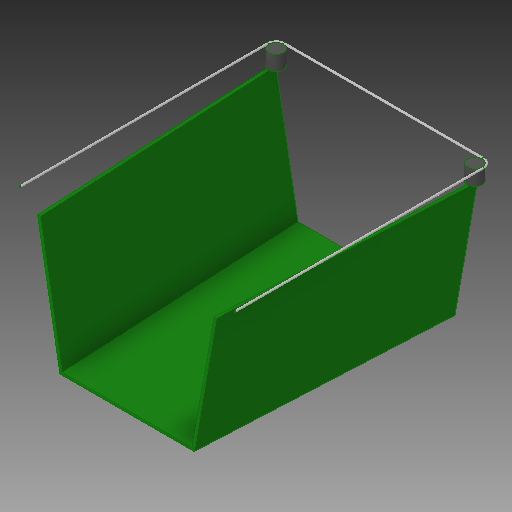
# Autodesk Inventor part: boat_segment
Saved by Autodesk Inventor 2019 (Build 230136000, 136)
## iProperties
Created: 2019-01-30
Part Number: boat_segment
Material: Generic
Document SubType Name: Modeling
Designer: suchanek
Density: 1 g/cm^3
Appearance: Default
boat_rim_angle: 80.00 deg
boat_width: 400.000 mm
boat_rim_thickness: 5.000 mm
boat_rim_plate_width: 0.000 mm
boat_part_length: 500.000 mm
boat_end_width: 350.000 mm
Author: suchanek
Autodesk Inventor part; units mm, degrees
ref_plane "YZ Plane" through (0, 0, 0) normal (1, 0, 0) x (0, 1, 0)
ref_plane "XZ Plane" through (0, 0, 0) normal (0, 1, 0) x (-1, 0, 0)
ref_plane "XY Plane" through (0, 0, 0) normal (0, 0, 1) x (1, 0, 0)
sketch "Sketch1" plane through (0, 0, 0) normal (0, 0, 1) x (1, 0, 0)
  line L0 (-160.1138, -255) -> (160.1138, -255)
  line L1 (200, 0) -> (155.9183, -250)
  line L2 (155.9183, -250) -> (-155.9183, -250)
  line L3 (-155.9183, -250) -> (-200, 0)
  line L4 (-160.1138, -255) -> (-204.1955, -5)
  line L5 (-204.1955, -5) -> (-204.1955, -5)
  line L6 (-204.1955, -5) -> (-205.0771, 0)
  line L7 (160.1138, -255) -> (204.1955, -5)
  line L8 (204.1955, -5) -> (204.1955, -5)
  line L9 (204.1955, -5) -> (205.0771, 0)
  line L10 (-205.0771, 0) -> (-200, 0)
  line L11 (200, 0) -> (205.0771, 0)
  line L12 (0, 0) -> (0, 16.0909)
  dimension "d0" = 5
  dimension "d1" = 5
  dimension "d2" = 5
  dimension "d3" = 0
  dimension "d4" = 0
  dimension "d5" = 400
  dimension "d6" = 250
  dimension "d7" = 80
  dimension "d8" = 80
  dimension "d9" = 5
  dimension "d10" = 5
  constraints: 26 end point, 4 horizontal, 3 collinear, 2 parallel, 1 horizontal alignment, 1 symmetric about line, 1 vertical
  measures "d0" distance between parallel lines of L2 L0
  measures "d1" distance between parallel lines of L7 L1
  measures "d2" distance between parallel lines of L3 L4
  measures "d3" distance between parallel lines of L4 L6
  measures "d4" distance between parallel lines of L7 L9
  measures "d5" distance of L1.start L3.end
  measures "d6" distance from line of L12.start L2
  measures "d7" angle of L3 L10
  measures "d8" angle of L11 L1
  measures "d9" distance between parallel lines of L11 L8
  measures "d10" distance between parallel lines of L10 L5
sketch "Sketch2" plane through (0, 0, 0) normal (1, 0, 0) x (0, 1, 0)
  line L0 (0, 0) -> (0, 500)
  dimension "d11" = 500
  constraints: 2 end point, 1 vertical
  measures "d11" distance of L0.start L0.end
ref_plane "Work Plane1" through (0, 0, 500) normal (0, 0, 1) x (1, 0, 0)
ref_plane "Work Plane2" through (-200, 0, 0) normal (0, -1, 0) x (-1, 0, 0)
sketch "Sketch5" plane through (-200, 0, 0) normal (0, -1, 0) x (-1, 0, 0)
  circle A0 centre (0, 0) radius 15
  line L0 (-360.1138, 0) -> (-404.1955, 0) projected
  circle A1 centre (-400, 0) radius 15
  line L1 (-400, 0) -> (-375, -500) projected
  point P0 (-200, 0)
  dimension "d34" = 30
  dimension "d35" = 30
  constraints: 2 centre point, 2 point on line, 1 coincident
  measures "d34" diameter of A0
  measures "d35" diameter of A1
extrude "Extrusion1" add sketch "Sketch5" against normal blind 30
sketch "Sketch6" plane through (-200, 30, 0) normal (0, 1, 0) x (1, 0, 0)
  line L0 (-17, -498.5563) -> (-17, 0)
  line L1 (44.0817, 0) -> (0, 0) projected
  arc A0 (0, 17) -> (-17, 0) centre (0, 0) ccw
  circle A1 centre (0, 0) radius 15 projected
  line L2 (0, 17) -> (400, 17)
  circle A2 centre (400, 0) radius 15 projected
  arc A3 (417, 0) -> (400, 17) centre (400, 0) ccw
  line L3 (417, 0) -> (417, -500)
  line L4 (400.3857, -500) -> (375, -500) projected
  point P0 (200, 0)
  dimension "d38" = 2
  constraints: 6 end point, 4 point on circle, 4 tangent, 2 centre point, 2 vertical, 1 coincident, 1 horizontal, 1 point on line
  measures "d38" radial gap between concentric circles of A0 A1
ref_plane "Work Plane3" through (-217, 30, 498.5563) normal (0, 0, -1) x (-1, 0, 0)
sketch "Sketch8" plane through (-217, 30, 498.5563) normal (0, 0, -1) x (-1, 0, 0)
  circle A0 centre (0, 0) radius 2
  point P0 (-217, -30)
  dimension "d40" = 4
  constraints: 1 centre point
  measures "d40" diameter of A0
sweep "Sweep1" add profiles "Sketch8" path "Sketch6" path curves L0 A0 L2 A3 L3
sketch "Sketch4" plane through (0, 0, 500) normal (0, 0, 1) x (1, 0, 0)
  line L0 (-135.1138, -255) -> (135.1138, -255)
  line L1 (175, 0) -> (130.9183, -250)
  line L2 (130.9183, -250) -> (-130.9183, -250)
  line L3 (-130.9183, -250) -> (-175, 0)
  line L4 (-135.1138, -255) -> (-179.1955, -5)
  line L5 (-179.1955, -5) -> (-180.0771, 0)
  line L6 (135.1138, -255) -> (179.1955, -5)
  line L7 (179.1955, -5) -> (180.0771, 0)
  line L8 (-180.0771, 0) -> (-175, 0)
  line L9 (175, 0) -> (180.0771, 0)
  line L10 (0, 0) -> (0, 12.0492)
  line L11 (-185, 30) -> (-215, 30) projected
  line L12 (-185, 30) -> (-185, 40)
  line L13 (215, 30) -> (185, 30) projected
  line L14 (185, 30) -> (185, 40)
  line L15 (-185, 0) -> (-215, 0) projected
  line L16 (-215, 0) -> (-232.122, 0)
  line L17 (-175, 0) -> (-175, 10.4521)
  point P0 (-200, 30)
  point P1 (200, 30)
  dimension "d12" = 5
  dimension "d13" = 5
  dimension "d14" = 5
  dimension "d15" = 0
  dimension "d16" = 0
  dimension "d17" = 350
  dimension "d18" = 250
  dimension "d19" = 80
  dimension "d20" = 80
  dimension "d21" = 5
  dimension "d22" = 5
  dimension "d47" = 10
  dimension "d48" = 10
  dimension "d49" = 0
  dimension "d50" = 25
  constraints: 30 end point, 4 vertical, 3 collinear, 3 horizontal, 2 coincident, 2 parallel, 1 horizontal alignment, 1 symmetric about line, 4 other
  measures "d12" distance between parallel lines of L2 L0
  measures "d13" distance between parallel lines of L6 L1
  measures "d14" distance between parallel lines of L3 L4
  measures "d15" distance between parallel lines of L4 L5
  measures "d16" distance between parallel lines of L6 L7
  measures "d17" distance of L1.start L3.end
  measures "d18" distance from line of L10.start L2
  measures "d19" angle of L3 L8
  measures "d20" angle of L9 L1
  measures "d47" distance of L11.start L12.end
  measures "d48" distance of L13.end L14.end
  measures "d49" distance between parallel lines of L8 L15
  measures "d50" distance from line of point (-200, 30) L17
loft "Loft2" add profiles "Sketch1", "Sketch4"
equation "\"d0\" = boat_rim_thickness"
equation "\"d1\" = boat_rim_thickness"
equation "\"d2\" = boat_rim_thickness"
equation "\"d5\" = boat_width"
equation "\"d7\" = boat_rim_angle"
equation "\"d8\" = boat_rim_angle"
equation "\"d9\" = boat_rim_thickness"
equation "\"d10\" = boat_rim_thickness"
equation "\"d11\" = boat_part_length"
equation "\"d12\" = d23"
equation "\"d13\" = d23"
equation "\"d14\" = d23"
equation "\"d17\" = boat_end_width"
equation "\"d19\" = d26"
equation "\"d20\" = d26"
equation "\"d21\" = d23"
equation "\"d22\" = d23"
equation "\"boat_rim_angle\" = 80deg"
equation "\"boat_width\" = 400"
equation "\"boat_rim_thickness\" = 5"
equation "\"boat_rim_plate_width\" = 0"
equation "\"boat_part_length\" = 500"
equation "\"boat_end_width\" = 350"
equation "\"d23\" = 5"
equation "\"d26\" = 80deg"
body "Solid1"
